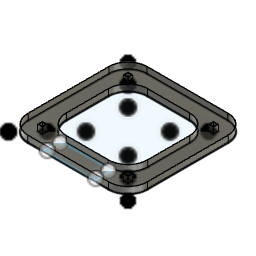
Unterseite-Outdoorwetter (Autodesk Fusion 360 design; units mm, degrees)
Autodesk Fusion 360 part; units mm, degrees
sketch "Skizze1" plane through (0, 0, 0) normal (0, 0, 1) x (1, 0, 0)
  line L0 (60, 0) -> (310, 0)
  line L1 (370, 60) -> (370, 310)
  line L2 (310, 370) -> (60, 370)
  line L3 (0, 310) -> (0, 60)
  line L4 (120, 60) -> (250, 60)
  line L5 (310, 120) -> (310, 250)
  line L6 (250, 310) -> (120, 310)
  line L7 (60, 250) -> (60, 120)
  arc A0 (120, 310) -> (60, 250) centre (120, 250) ccw
  arc A1 (310, 250) -> (250, 310) centre (250, 250) ccw
  arc A2 (250, 60) -> (310, 120) centre (250, 120) ccw
  arc A3 (60, 120) -> (120, 60) centre (120, 120) ccw
  arc A4 (310, 0) -> (370, 60) centre (310, 60) ccw
  arc A5 (0, 60) -> (60, 0) centre (60, 60) ccw
  arc A6 (60, 370) -> (0, 310) centre (60, 310) ccw
  arc A7 (370, 310) -> (310, 370) centre (310, 310) ccw
  line L8 (368.5, 60) -> (368.5, 310)
  arc A8 (368.5, 310) -> (310, 368.5) centre (310, 310) ccw
  line L9 (310, 368.5) -> (60, 368.5)
  arc A9 (60, 368.5) -> (1.5, 310) centre (60, 310) ccw
  line L10 (1.5, 310) -> (1.5, 60)
  arc A10 (1.5, 60) -> (60, 1.5) centre (60, 60) ccw
  line L11 (60, 1.5) -> (310, 1.5)
  arc A11 (310, 1.5) -> (368.5, 60) centre (310, 60) ccw
  line L12 (120, 58.5) -> (250, 58.5)
  arc A12 (250, 58.5) -> (311.5, 120) centre (250, 120) ccw
  line L13 (311.5, 120) -> (311.5, 250)
  arc A13 (311.5, 250) -> (250, 311.5) centre (250, 250) ccw
  line L14 (250, 311.5) -> (120, 311.5)
  arc A14 (120, 311.5) -> (58.5, 250) centre (120, 250) ccw
  line L15 (58.5, 250) -> (58.5, 120)
  arc A15 (58.5, 120) -> (120, 58.5) centre (120, 120) ccw
  line L16 (105, 5) -> (265, 5)
  line L17 (265, 5) -> (265, 55)
  line L18 (265, 55) -> (105, 55)
  line L19 (105, 55) -> (105, 5)
  line L20 (310, 60) -> (325, 60)
  line L21 (325, 60) -> (325, 45)
  line L22 (325, 45) -> (310, 45)
  line L23 (310, 45) -> (310, 60)
  line L24 (312.5, 57.5) -> (322.5, 57.5)
  line L25 (322.5, 57.5) -> (322.5, 47.5)
  line L26 (322.5, 47.5) -> (312.5, 47.5)
  line L27 (312.5, 47.5) -> (312.5, 57.5)
  line L28 (310, 310) -> (325, 310)
  line L29 (325, 310) -> (325, 325)
  line L30 (325, 325) -> (310, 325)
  line L31 (310, 325) -> (310, 310)
  line L32 (60, 310) -> (45, 310)
  line L33 (45, 310) -> (45, 325)
  line L34 (45, 325) -> (60, 325)
  line L35 (60, 325) -> (60, 310)
  line L36 (57.5, 312.5) -> (47.5, 312.5)
  line L37 (47.5, 312.5) -> (47.5, 322.5)
  line L38 (47.5, 322.5) -> (57.5, 322.5)
  line L39 (57.5, 322.5) -> (57.5, 312.5)
  line L40 (322.5, 312.5) -> (322.5, 322.5)
  line L41 (322.5, 322.5) -> (312.5, 322.5)
  line L42 (312.5, 322.5) -> (312.5, 312.5)
  line L43 (312.5, 312.5) -> (322.5, 312.5)
  line L44 (60, 60) -> (45, 60)
  line L45 (45, 60) -> (45, 45)
  line L46 (45, 45) -> (60, 45)
  line L47 (60, 45) -> (60, 60)
  line L48 (47.5, 47.5) -> (57.5, 47.5)
  line L49 (57.5, 47.5) -> (57.5, 57.5)
  line L50 (57.5, 57.5) -> (47.5, 57.5)
  line L51 (47.5, 57.5) -> (47.5, 47.5)
  circle A16 centre (110, 50) radius 5
  circle A17 centre (110, 10) radius 5
  circle A18 centre (260, 50) radius 5
  circle A19 centre (260, 10) radius 5
  point P0 (370, 0)
  point P1 (0, 370)
  dimension "d3" = 370
  dimension "d4" = 370
  dimension "d6" = 60
  dimension "d7" = -1.5
  dimension "d8" = 1.5
  dimension "d11" = 160
  dimension "d12" = 50
  dimension "d13" = 15
  dimension "d14" = 15
  dimension "d15" = 2.5
  dimension "d16" = 15
  dimension "d17" = 15
  dimension "d18" = 15
  dimension "d19" = 15
  dimension "d20" = 2.5
  dimension "d21" = -2.5
  dimension "d22" = 15
  dimension "d23" = 15
  dimension "d24" = -2.5
  dimension "d35" = 10
  dimension "d36" = 10
  dimension "d37" = 10
  dimension "d38" = 10
  constraint horizontal L0
  constraint vertical L1
  constraint horizontal L2
  constraint vertical L3
  constraint tangent L6 A0
  constraint tangent L7 A0
  constraint tangent L5 A1
  constraint tangent L6 A1
  constraint equal A0 A1
  constraint tangent L4 A2
  constraint tangent L5 A2
  constraint equal A0 A2
  constraint tangent L4 A3
  constraint tangent L7 A3
  constraint equal A0 A3
  constraint coincident P0 L0
  constraint coincident P0 L1
  constraint tangent L0 A4
  constraint tangent L1 A4
  constraint equal A0 A4
  constraint coincident origin L0
  constraint coincident origin L3
  constraint tangent L0 A5
  constraint tangent L3 A5
  constraint equal A0 A5
  constraint coincident P1 L2
  constraint coincident P1 L3
  constraint tangent L2 A6
  constraint tangent L3 A6
  constraint equal A0 A6
  constraint tangent L1 A7
  constraint tangent L2 A7
  constraint equal A0 A7
  constraint horizontal L16
  constraint vertical L17
  constraint horizontal L18
  constraint vertical L19
  constraint horizontal L20
  constraint vertical L21
  constraint horizontal L22
  constraint vertical L23
  constraint coincident A4.centre A11.centre
  constraint horizontal L28
  constraint vertical L29
  constraint horizontal L30
  constraint vertical L31
  constraint coincident A7.centre A8.centre
  constraint horizontal L32
  constraint vertical L33
  constraint horizontal L34
  constraint vertical L35
  constraint coincident A6.centre A9.centre
  constraint horizontal L44
  constraint vertical L45
  constraint horizontal L46
  constraint vertical L47
  constraint coincident A5.centre A10.centre
  measures "d3" distance of origin P0
  measures "d4" distance of origin P1
  measures "d6" radius of A0
  measures "d11" distance of L16.start L16.end
  measures "d12" distance of L16.start L18.end
  measures "d13" distance of A4.centre L20.end
  measures "d14" distance of A4.centre L22.end
  measures "d16" distance of A7.centre L28.end
  measures "d17" distance of A7.centre L30.end
  measures "d18" distance of A6.centre L32.end A4.centre
  measures "d19" distance of A6.centre L34.end A4.centre
  measures "d22" distance of A5.centre L44.end
  measures "d23" distance of A5.centre L46.end
  measures "d35" diameter of A16
  measures "d36" diameter of A17
  measures "d37" diameter of A18
  measures "d38" diameter of A19
extrude "Extrusion1" add sketch "Skizze1" along normal blind 2 contours L16 L19 A17 | L16 L17 L18 L19 A16 A17 A18 A19 | A17 | L16 L17 A19 | A19 | L18 L19 A16 | A16 | L17 L18 A18 | A18 | L20 L21 L22 L23 | L24 L25 L26 L27 | L28 L29 L30 L31 | L32 L33 L34 L35 | L36 L37 L38 L39 | L40 L41 L42 L43 | L44 L45 L46 L47 | L48 L49 L50 L51 makes body 1 at (50, 55, 0) makes body 2 at (315, 55, 0) makes body 3 at (55, 315, 0) makes body 4 at (158.3333, 38.3333, 0) makes body 5 at (315, 320, 0)
extrude "Extrusion2" add sketch "Skizze1" along normal blind 2 contours L8 A8 L9 A9 L10 A10 L11 A11 bodies 1 2 3 4 5
extrude "Extrusion3" add sketch "Skizze1" along normal blind 20 contours L0 L1 L2 L3 A4 A5 A6 A7 | L12 A12 L13 A13 L14 A14 L15 A15 bodies 1
extrude "Extrusion4" add sketch "Skizze1" along normal blind 2 separate body contours L24 L25 L26 L27 | L36 L37 L38 L39 | L40 L41 L42 L43 | L48 L49 L50 L51 makes body 6 at (319.1667, 315.8333, 0) makes body 7 at (50.8333, 54.1667, 0) makes body 8 at (54.1667, 315.8333, 0) makes body 9 at (315.8333, 54.1667, 0)
extrude "Extrusion5" add sketch "Skizze1" along normal blind 20 contours L20 L21 L22 L23 | L28 L29 L30 L31 | L32 L33 L34 L35 | L44 L45 L46 L47 bodies 1 6 7 8 9
